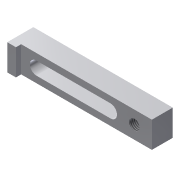
# Autodesk Inventor part: LabClamp
Saved by Autodesk Inventor 2015 (Build 190159000, 159)
## iProperties
Created: 2015-03-27
Part Number: LabClamp
Material: Generic
Document SubType Name: Modeling
Designer: jad211
Density: 1 g/cm^3
Appearance: Aluminum - Flat
Author: jad211
Autodesk Inventor part; units mm, degrees
ref_plane "YZ Plane" through (0, 0, 0) normal (1, 0, 0) x (0, 1, 0)
ref_plane "XZ Plane" through (0, 0, 0) normal (0, 1, 0) x (-1, 0, 0)
ref_plane "XY Plane" through (0, 0, 0) normal (0, 0, 1) x (1, 0, 0)
sketch "Sketch1" plane through (0, 0, 0) normal (0, 1, 0) x (-1, 0, 0)
  line L0 (-40, 7.5) -> (40, 7.5)
  line L1 (40, 7.5) -> (40, -7.5)
  line L2 (40, -7.5) -> (-40, -7.5)
  line L3 (-40, -7.5) -> (-40, 7.5)
  line L4 (-40, 7.5) -> (40, -7.5) construction
  line L5 (40, 7.5) -> (-40, -7.5) construction
  line L6 (30, 0) -> (-20, 0) construction
  line L7 (26.25, 3.75) -> (-16.25, 3.75)
  line L8 (-16.25, -3.75) -> (26.25, -3.75)
  arc A0 (26.25, -3.75) -> (26.25, 3.75) centre (26.25, 0) ccw
  arc A1 (-16.25, 3.75) -> (-16.25, -3.75) centre (-16.25, 0) ccw
  point P0 (0, 0)
  point P1 (5, 0)
  dimension "d0" = 15
  dimension "d1" = 80
  dimension "d2" = 7.5
  dimension "d3" = 50
  dimension "d4" = 10
  constraints: 20 end point, 6 point on circle, 4 parallel, 4 tangent, 3 midpoint, 2 centre point, 2 point on line, 1 horizontal, 1 perpendicular
  measures "d0" distance of L0.end L1.end
  measures "d1" distance of L1.end L2.end
  measures "d2" distance between parallel lines of L8 L7
  measures "d3" distance of L6.end L6.start
  measures "d4" distance from line of L1 L6.start
extrude "Extrusion1" add sketch "Sketch1" along normal blind 12
sketch "Sketch2" plane through (0, 0, 0) normal (0, -1, 0) x (1, 0, 0)
  line L0 (-40, 7.5) -> (-35, 7.5)
  line L1 (-35, 7.5) -> (-35, -7.5)
  line L2 (-35, -7.5) -> (-40, -7.5)
  line L3 (-40, -7.5) -> (-40, 7.5)
  point P0 (0, 0)
  dimension "d7" = 5
  constraints: 8 end point, 2 parallel, 1 horizontal, 1 perpendicular
  measures "d7" distance of L1.end L2.end
extrude "Extrusion2" add sketch "Sketch2" along normal blind 3
sketch "Sketch3" plane through (0, 12, 0) normal (0, 1, 0) x (1, 0, 0)
  circle A0 centre (30, 0) radius 3
  line L0 (40, -7.5) -> (40, 7.5) projected
  point P0 (0, 0)
  dimension "d19" = 6
  dimension "d20" = 10
  constraints: 1 centre point
  measures "d19" diameter of A0
  measures "d20" distance from line of L0 A0.centre
extrude "Extrusion3" cut sketch "Sketch3" against normal up to next
thread "Thread1" size "M6x1" class "6H" standard "ANSI Metric M Profile" full length
body "Solid1"
